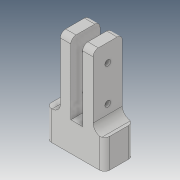
# Autodesk Inventor part: acrylicMount
Saved by Autodesk Inventor 2018 (Build 220112000, 112)
## iProperties
Created: 2020-02-23
Part Number: acrylicMount
Material: Generic
Document SubType Name: Modeling
Designer: anirudh
Density: 1 g/cm^3
Appearance: Default
Author: anirudh
Autodesk Inventor part; units mm, degrees
ref_plane "YZ Plane" through (0, 0, 0) normal (1, 0, 0) x (0, 1, 0)
ref_plane "XZ Plane" through (0, 0, 0) normal (0, 1, 0) x (-1, 0, 0)
ref_plane "XY Plane" through (0, 0, 0) normal (0, 0, 1) x (1, 0, 0)
sketch "Sketch1" plane through (0, 0, 0) normal (0, 1, 0) x (-1, 0, 0)
  line L0 (0, 0) -> (35.56, 0)
  line L1 (35.56, 0) -> (35.56, -17.78)
  line L2 (35.56, -17.78) -> (0, -17.78)
  line L3 (0, -17.78) -> (0, 0)
  dimension "d0" = 35.56
  dimension "d1" = 17.78
  constraints: 8 end point, 2 parallel, 1 horizontal, 1 perpendicular
  measures "d0" distance of L1.end L2.end
  measures "d1" distance of L0.end L1.end
extrude "Extrusion1" add sketch "Sketch1" along normal blind 60.96
sketch "Sketch2" plane through (0, 0, 0) normal (0, -1, 0) x (1, 0, 0)
  line L0 (-35.56, 0) -> (0, 0) projected
  line L1 (0, -17.78) -> (-35.56, -17.78) projected
  line L2 (0, 0) -> (0, -17.78) projected
  line L3 (-35.56, -17.78) -> (-35.56, 0) projected
  circle A0 centre (-8.89, -8.89) radius 2.1971
  circle A1 centre (-26.67, -8.89) radius 2.1971
  dimension "d4" = 4.3942
  dimension "d5" = 4.3942
  constraints: 2 centre point
  measures "d4" diameter of A0
  measures "d5" diameter of A1
extrude "Extrusion2" cut sketch "Sketch2" against normal blind 4.8006 contours A0 | A1
sketch "Sketch3" plane through (0, 60.96, 0) normal (0, 1, 0) x (1, 0, 0)
  line L0 (-17.78, 0) -> (-20.574, 0)
  line L1 (-20.574, 0) -> (-14.986, 0)
  line L2 (-14.986, 0) -> (-14.986, 17.78)
  line L3 (-14.986, 17.78) -> (-20.574, 17.78)
  line L4 (-20.574, 17.78) -> (-20.574, 0)
  point P0 (0, 0)
  point P1 (-35.56, 0)
  dimension "d9" = 5.588
  constraints: 10 end point, 2 parallel, 1 horizontal, 1 perpendicular
  measures "d9" distance of L3.end L2.end
extrude "Extrusion3" cut sketch "Sketch3" against normal blind 43.1292
sketch "Sketch4" plane through (0, 60.96, 0) normal (0, 1, 0) x (1, 0, 0)
  line L0 (-14.986, 17.78) -> (-14.986, 0) projected
  line L1 (-14.986, 0) -> (0, 0) projected
  line L2 (-20.574, 0) -> (-20.574, 17.78) projected
  line L3 (-35.56, 0) -> (-20.574, 0) projected
  line L4 (-35.56, 17.78) -> (0, 17.78) projected
  line L5 (-26.924, 0) -> (-35.56, 0)
  line L6 (-35.56, 0) -> (-35.56, 17.78)
  line L7 (-35.56, 17.78) -> (-26.924, 17.78)
  line L8 (-26.924, 17.78) -> (-26.924, 0)
  line L9 (0, 0) -> (0, 17.78) projected
  line L10 (-8.636, 0) -> (0, 0)
  line L11 (0, 0) -> (0, 17.78)
  line L12 (0, 17.78) -> (-8.636, 17.78)
  line L13 (-8.636, 17.78) -> (-8.636, 0)
  dimension "d12" = 6.35
  dimension "d13" = 6.35
  constraints: 16 end point, 4 parallel, 2 horizontal, 2 perpendicular, 2 point on line
  measures "d12" distance of L0.end L10.start
  measures "d13" distance of L2.start L5.start
extrude "Extrusion4" cut sketch "Sketch4" against normal blind 43.1292 contours L4 L9 L1 L13 | L3 L6 L4 L8
sketch "Sketch5" plane through (-8.636, 60.96, 0) normal (1, 0, 0) x (0, 0, -1)
  line L0 (0, 0) -> (0, -43.1292) projected
  line L1 (17.78, -43.1292) -> (17.78, 0) projected
  line L2 (0, -43.1292) -> (17.78, -43.1292)
  line L3 (0, -43.1292) -> (17.78, -43.1292) projected
  line L4 (17.78, 0) -> (0, 0) projected
  circle A0 centre (8.89, -10.7823) radius 1.75
  circle A1 centre (8.89, -32.3469) radius 1.75
  point P0 (0, -60.96)
  dimension "d16" = 3.5
  dimension "d17" = 3.5
  constraints: 2 centre point, 2 end point, 1 horizontal
  measures "d16" diameter of A0
  measures "d17" diameter of A1
extrude "Extrusion5" cut sketch "Sketch5" against normal blind 43.1292 contours A0 | A1
sketch "Sketch6" plane through (0, 60.96, 0) normal (0, 1, 0) x (1, 0, 0)
  line L0 (-14.986, 17.78) -> (-14.986, 0) projected
  line L1 (-35.56, 17.78) -> (0, 17.78) projected
  line L2 (-14.986, 0) -> (-13.335, 0)
  line L3 (-13.335, 0) -> (-13.335, 17.78)
  line L4 (-13.335, 17.78) -> (-14.986, 17.78)
  line L5 (-14.986, 17.78) -> (-14.986, 0)
  point P0 (0, 0)
  dimension "d22" = 1.651
  constraints: 8 end point, 2 parallel, 1 horizontal, 1 perpendicular, 1 point on line
  measures "d22" distance of L4.end L3.end
extrude "Extrusion6" cut sketch "Sketch6" against normal blind 43.1292
sketch "Sketch7" plane through (-8.636, 60.96, 0) normal (1, 0, 0) x (0, 0, -1)
  line L0 (0, 0) -> (0, -43.1292) projected
  line L1 (0, -43.1292) -> (17.78, -43.1292) projected
  line L2 (0, 0) -> (17.78, 0)
  line L3 (17.78, 0) -> (17.78, -43.1292)
  line L4 (17.78, -43.1292) -> (0, -43.1292)
  line L5 (0, -43.1292) -> (0, 0)
  circle A0 centre (8.89, -10.7823) radius 1.75 projected
  circle A1 centre (8.89, -10.7823) radius 1.75
  circle A2 centre (8.89, -32.3469) radius 1.75 projected
  circle A3 centre (8.89, -32.3469) radius 1.75
  point P0 (0, -60.96)
  constraints: 8 end point, 2 centre point, 2 coincident, 2 parallel, 1 horizontal, 1 perpendicular
extrude "Extrusion7" add sketch "Sketch7" along normal blind 1.651
fillet "Fillet3" radius 5.08 2 edges at (-6.985, 17.8308, -8.89) (-26.924, 17.8308, -8.89)
fillet "Fillet4" radius 3.175 8 edges at (0, 8.9154, 0) (0, 8.9154, -17.78) (-35.56, 8.9154, -17.78) (-10.16, 60.96, 0) (-23.749, 60.96, 0) (-10.16, 60.96, -17.78) (-23.749, 60.96, -17.78) (-35.56, 8.9154, 0)
body "Solid1"
